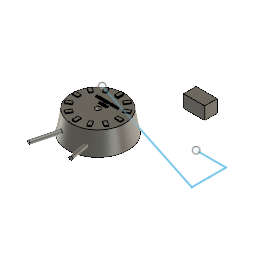
AlarmClock v1 (Autodesk Fusion 360 design; units mm, degrees)
Autodesk Fusion 360 part; units mm, degrees
(part 1 of 2)
sketch "Sketch1" plane through (0, 0, 0) normal (0, 0, 1) x (1, 0, 0)
  circle A0 centre (0, 0) radius 70.7107
  constraint coincident A0.centre origin
extrude "Extrude1" add sketch "Sketch1" along normal blind 50 draft -10 makes body 1
sketch "Sketch2" plane through (0, 0, 50) normal (0, 0, 1) x (-1, 0, 0)
  circle A0 centre (0, 0) radius 61.8943
  line L0 (3.9578, -43.206) -> (-3.9578, -43.206)
  line L1 (-3.9578, -43.206) -> (-3.9578, -56.794)
  line L2 (-3.9578, -56.794) -> (3.9578, -56.794)
  line L3 (3.9578, -56.794) -> (3.9578, -43.206)
  line L4 (3.9578, -43.206) -> (-3.9578, -56.794) construction
  line L5 (-3.9578, -43.206) -> (3.9578, -56.794) construction
  point P0 (0, -50)
  constraint horizontal L0
  constraint perpendicular L0 L1
  constraint parallel L0 L2
  constraint parallel L1 L3
  constraint coincident L4 P0
  constraint coincident L5 P0
extrude "Extrude2" add sketch "Sketch2" along normal blind 2 contours L0 L1 L2 L3 bodies 1
extrude "Extrude3" add 1 faces at (1.3193, 47.7353, 52) along direction (0, 0, 1) blind 2 separate body on bodies 1 makes body 2
pattern_circular "C-Pattern1" count 12 over 360 about axis through (0, 0, 1.75) along (0, 0, 1) of bodies 2 makes body 3 at (-24.9898, 45.9222, 52) makes body 4 at (-41.9996, 22.7251, 52) makes body 5 at (-47.7353, 1.3193, 52) makes body 6 at (-40.6804, -25.0102, 52) makes body 7 at (-25.0102, -40.6804, 52) makes body 8 at (-1.3193, -47.7353, 52) makes body 9 at (22.7251, -41.9996, 52) makes body 10 at (40.6804, -25.0102, 52) makes body 11 at (47.7353, -1.3193, 52) makes body 12 at (41.9996, 22.7251, 52) makes body 13 at (25.0102, 40.6804, 52)
sketch "Sketch3" plane through (0, 0, 50) normal (0, 0, 1) x (-1, 0, 0)
  line L0 (3.9578, -56.794) -> (-3.9578, -56.794)
  line L1 (-3.9578, -56.794) -> (-3.9578, -43.206)
  line L2 (-3.9578, -43.206) -> (3.9578, -43.206)
  line L3 (3.9578, -43.206) -> (3.9578, -56.794)
  circle A0 centre (0, 0) radius 61.8943
  circle A1 centre (0, 0) radius 6.2665
  constraint coincident A0.centre A1.centre
extrude "Extrude4" cut sketch "Sketch3" against normal blind 30 contours A1 bodies 1
sketch "Sketch4" plane through (0, 0, 50) normal (0, 0, 1) x (-1, 0, 0)
  circle A0 centre (0, 0) radius 6.2665
  line L0 (3.9578, -56.794) -> (-3.9578, -56.794)
  line L1 (-3.9578, -56.794) -> (-3.9578, -43.206)
  line L2 (-3.9578, -43.206) -> (3.9578, -43.206)
  line L3 (3.9578, -43.206) -> (3.9578, -56.794)
  circle A1 centre (0, 0) radius 61.8943
  line L4 (20, -10) -> (-20, -10)
  dimension "d12" = 5
  dimension "d13" = 5
  text T0 "NGUYEN VAN A" font "Arial" height 5 align centre spacing 1 along the path letters at x, y, angle (26.4137, -26.3233, 180) (21.3694, -26.3233, 180) (15.9362, -26.3233, 180) (10.8919, -26.3233, 180) (6.2329, -26.3233, 180) (1.574, -26.3233, 180) (-3.4703, -26.3233, 180) (-5.411, -26.3233, 180) (-10.0699, -26.3233, 180) (-14.7493, -26.3233, 180) (-19.7937, -26.3233, 180) (-21.7343, -26.3233, 180)
  text T1 "MSSV" font "Arial" height 5 align centre spacing 1 along the path L4 letters at x, y, angle (9.8977, -16.3233, 180) (4.0791, -16.3233, 180) (-0.5798, -16.3233, 180) (-5.2387, -16.3233, 180)
  constraint horizontal L4
extrude "Extrude5" add sketch "Sketch4" along normal blind 2 text T0 T1 bodies 1
sketch "Sketch5" plane through (0, 0, 50) normal (0, 0, 1) x (-1, 0, 0)
  line L0 (9.3793, -10) -> (9.3793, -15)
  line L1 (9.3793, -15) -> (8.3834, -15)
  line L2 (8.3834, -15) -> (7.1999, -11.4598)
  spline S0 degree 3 poles (7.1999, -11.4598) (7.1522, -11.3158) (7.0708, -11.0697) (6.9933, -10.8223) (6.9611, -10.7196) knots 0 0 0 0 0.045488 0.077767 0.077767 0.077767 0.077767
  spline S1 degree 3 poles (6.9611, -10.7196) (6.925, -10.832) (6.8389, -11.1) (6.7479, -11.3664) (6.6951, -11.5211) knots 0 0 0 0 0.035404 0.084451 0.084451 0.084451 0.084451
  line L3 (6.6951, -11.5211) -> (5.498, -15)
  line L4 (5.498, -15) -> (4.6078, -15)
  line L5 (4.6078, -15) -> (4.6078, -10)
  line L6 (4.6078, -10) -> (5.2456, -10)
  line L7 (5.2456, -10) -> (5.2456, -14.1849)
  line L8 (5.2456, -14.1849) -> (6.6985, -10)
  line L9 (6.6985, -10) -> (7.2954, -10)
  line L10 (7.2954, -10) -> (8.7415, -14.2565)
  line L11 (8.7415, -14.2565) -> (8.7415, -10)
  line L12 (8.7415, -10) -> (9.3793, -10)
  line L13 (-7.2067, -10) -> (-5.2694, -15)
  line L14 (-5.2694, -15) -> (-5.9857, -15)
  line L15 (-5.9857, -15) -> (-7.2851, -11.3677)
  spline S2 degree 3 poles (-7.2851, -11.3677) (-7.3345, -11.2271) (-7.4296, -10.9567) (-7.5094, -10.6814) (-7.5477, -10.5491) knots 0 0 0 0 0.04468 0.08598 0.08598 0.08598 0.08598
  spline S3 degree 3 poles (-7.5477, -10.5491) (-7.5881, -10.686) (-7.6695, -10.9616) (-7.7677, -11.2317) (-7.8172, -11.3677) knots 0 0 0 0 0.042804 0.086194 0.086194 0.086194 0.086194
  line L16 (-7.8172, -11.3677) -> (-9.1678, -15)
  line L17 (-9.1678, -15) -> (-9.8431, -15)
  line L18 (-9.8431, -15) -> (-7.8854, -10)
  line L19 (-7.8854, -10) -> (-7.2067, -10)
  line L20 (25.8817, -20) -> (25.8817, -25)
  line L21 (25.8817, -25) -> (25.2029, -25)
  line L22 (25.2029, -25) -> (22.5767, -21.0744)
  line L23 (22.5767, -21.0744) -> (22.5767, -25)
  line L24 (22.5767, -25) -> (21.9424, -25)
  line L25 (21.9424, -25) -> (21.9424, -20)
  line L26 (21.9424, -20) -> (22.6211, -20)
  line L27 (22.6211, -20) -> (25.2473, -23.9291)
  line L28 (25.2473, -23.9291) -> (25.2473, -20)
  line L29 (25.2473, -20) -> (25.8817, -20)
  line L30 (5.6804, -20) -> (5.6804, -25)
  line L31 (5.6804, -25) -> (2.0651, -25)
  line L32 (2.0651, -25) -> (2.0651, -24.41)
  line L33 (2.0651, -24.41) -> (5.0188, -24.41)
  line L34 (5.0188, -24.41) -> (5.0188, -22.8786)
  line L35 (5.0188, -22.8786) -> (2.2527, -22.8786)
  line L36 (2.2527, -22.8786) -> (2.2527, -22.292)
  line L37 (2.2527, -22.292) -> (5.0188, -22.292)
  line L38 (5.0188, -22.292) -> (5.0188, -20.59)
  line L39 (5.0188, -20.59) -> (1.9492, -20.59)
  line L40 (1.9492, -20.59) -> (1.9492, -20)
  line L41 (1.9492, -20) -> (5.6804, -20)
  line L42 (-15.2814, -20) -> (-15.2814, -25)
  line L43 (-15.2814, -25) -> (-15.9601, -25)
  line L44 (-15.9601, -25) -> (-18.5863, -21.0744)
  line L45 (-18.5863, -21.0744) -> (-18.5863, -25)
  line L46 (-18.5863, -25) -> (-19.2207, -25)
  line L47 (-19.2207, -25) -> (-19.2207, -20)
  line L48 (-19.2207, -20) -> (-18.542, -20)
  line L49 (-18.542, -20) -> (-15.9158, -23.9291)
  line L50 (-15.9158, -23.9291) -> (-15.9158, -20)
  line L51 (-15.9158, -20) -> (-15.2814, -20)
  line L52 (-21.7241, -20) -> (-23.6443, -25)
  line L53 (-23.6443, -25) -> (-24.3571, -25)
  line L54 (-24.3571, -25) -> (-26.4035, -20)
  line L55 (-26.4035, -20) -> (-25.6497, -20)
  line L56 (-25.6497, -20) -> (-25.0665, -21.5143)
  line L57 (-25.0665, -21.5143) -> (-22.9758, -21.5143)
  line L58 (-22.9758, -21.5143) -> (-22.4267, -20)
  line L59 (-22.4267, -20) -> (-21.7241, -20)
  line L60 (-7.3789, -20) -> (-5.4417, -25)
  line L61 (-5.4417, -25) -> (-6.1579, -25)
  line L62 (-6.1579, -25) -> (-7.4574, -21.3677)
  spline S4 degree 3 poles (-7.4574, -21.3677) (-7.5068, -21.2271) (-7.6019, -20.9567) (-7.6817, -20.6814) (-7.72, -20.5491) knots 0 0 0 0 0.04468 0.08598 0.08598 0.08598 0.08598
  spline S5 degree 3 poles (-7.72, -20.5491) (-7.7604, -20.686) (-7.8417, -20.9616) (-7.94, -21.2317) (-7.9894, -21.3677) knots 0 0 0 0 0.042804 0.086194 0.086194 0.086194 0.086194
  line L63 (-7.9894, -21.3677) -> (-9.34, -25)
  line L64 (-9.34, -25) -> (-10.0153, -25)
  line L65 (-10.0153, -25) -> (-8.0576, -20)
  line L66 (-8.0576, -20) -> (-7.3789, -20)
  line L67 (12.1163, -25) -> (11.4546, -25)
  line L68 (11.4546, -25) -> (11.4546, -22.1112)
  spline S6 degree 3 poles (11.4546, -22.1112) (11.4578, -21.8841) (11.4634, -21.4772) (11.5756, -21.0866) (11.6252, -20.9141) knots 0 0 0 0 0.06775 0.121395 0.121395 0.121395 0.121395
  spline S7 degree 3 poles (11.6252, -20.9141) (11.6954, -20.772) (11.8396, -20.48) (12.1047, -20.2902) (12.2408, -20.1927) knots 0 0 0 0 0.046779 0.096143 0.096143 0.096143 0.096143
  spline S8 degree 3 poles (12.2408, -20.1927) (12.4095, -20.1118) (12.7778, -19.9351) (13.1871, -19.9219) (13.4089, -19.9147) knots 0 0 0 0 0.055521 0.121246 0.121246 0.121246 0.121246
  spline S9 degree 3 poles (13.4089, -19.9147) (13.6249, -19.921) (14.0234, -19.9325) (14.3903, -20.0864) (14.5583, -20.1569) knots 0 0 0 0 0.064151 0.118358 0.118358 0.118358 0.118358
  spline S10 degree 3 poles (14.5583, -20.1569) (14.6964, -20.2462) (14.9709, -20.4236) (15.1213, -20.7136) (15.1961, -20.8578) knots 0 0 0 0 0.048411 0.096232 0.096232 0.096232 0.096232
  spline S11 degree 3 poles (15.1961, -20.8578) (15.2516, -21.0374) (15.3776, -21.445) (15.3837, -21.8722) (15.3871, -22.1112) knots 0 0 0 0 0.05613 0.12736 0.12736 0.12736 0.12736
  line L69 (15.3871, -22.1112) -> (15.3871, -25)
  line L70 (15.3871, -25) -> (14.7254, -25)
  line L71 (14.7254, -25) -> (14.7254, -22.1146)
  spline S12 degree 3 poles (14.7254, -22.1146) (14.7248, -21.9247) (14.7236, -21.5991) (14.6394, -21.2853) (14.6044, -21.1545) knots 0 0 0 0 0.056655 0.097122 0.097122 0.097122 0.097122
  spline S13 degree 3 poles (14.6044, -21.1545) (14.5565, -21.0573) (14.4601, -20.8618) (14.2792, -20.74) (14.1883, -20.6787) knots 0 0 0 0 0.0319 0.064192 0.064192 0.064192 0.064192
  spline S14 degree 3 poles (14.1883, -20.6787) (14.0806, -20.63) (13.8517, -20.5264) (13.6002, -20.5167) (13.4669, -20.5116) knots 0 0 0 0 0.035099 0.074671 0.074671 0.074671 0.074671
  spline S15 degree 3 poles (13.4669, -20.5116) (13.2507, -20.5165) (12.8685, -20.5251) (12.5604, -20.7464) (12.4267, -20.8424) knots 0 0 0 0 0.063045 0.111418 0.111418 0.111418 0.111418
  spline S16 degree 3 poles (12.4267, -20.8424) (12.337, -21.0002) (12.1147, -21.3909) (12.1157, -21.8443) (12.1163, -22.1146) knots 0 0 0 0 0.053658 0.13291 0.13291 0.13291 0.13291
  line L72 (12.1163, -22.1146) -> (12.1163, -25)
  line L73 (3.7653, -11.6064) -> (3.1412, -11.661)
  spline S17 degree 3 poles (3.1412, -11.661) (3.1236, -11.5447) (3.0906, -11.3272) (2.9844, -11.1349) (2.9349, -11.0454) knots 0 0 0 0 0.034936 0.065388 0.065388 0.065388 0.065388
  spline S18 degree 3 poles (2.9349, -11.0454) (2.8701, -10.9677) (2.7313, -10.8013) (2.5359, -10.7069) (2.4318, -10.6565) knots 0 0 0 0 0.030005 0.064234 0.064234 0.064234 0.064234
  spline S19 degree 3 poles (2.4318, -10.6565) (2.3122, -10.6133) (2.0643, -10.5236) (1.8008, -10.5135) (1.6644, -10.5082) knots 0 0 0 0 0.037908 0.078579 0.078579 0.078579 0.078579
  spline S20 degree 3 poles (1.6644, -10.5082) (1.5446, -10.5119) (1.3165, -10.5188) (1.0991, -10.5879) (0.9959, -10.6207) knots 0 0 0 0 0.035752 0.068081 0.068081 0.068081 0.068081
  spline S21 degree 3 poles (0.9959, -10.6207) (0.9073, -10.6593) (0.7411, -10.7316) (0.6207, -10.8664) (0.5645, -10.9294) knots 0 0 0 0 0.028587 0.053609 0.053609 0.053609 0.053609
  spline S22 degree 3 poles (0.5645, -10.9294) (0.5232, -10.9958) (0.4415, -11.1272) (0.4291, -11.2813) (0.4229, -11.3574) knots 0 0 0 0 0.023091 0.045667 0.045667 0.045667 0.045667
  spline S23 degree 3 poles (0.4229, -11.3574) (0.4282, -11.4329) (0.4387, -11.5816) (0.5196, -11.7068) (0.5593, -11.7684) knots 0 0 0 0 0.022304 0.043934 0.043934 0.043934 0.043934
  spline S24 degree 3 poles (0.5593, -11.7684) (0.6169, -11.8263) (0.7458, -11.9559) (0.9156, -12.0251) (1.0095, -12.0634) knots 0 0 0 0 0.024245 0.054313 0.054313 0.054313 0.054313
  spline S25 degree 3 poles (1.0095, -12.0634) (1.117, -12.0979) (1.4101, -12.1919) (1.7098, -12.2625) (1.8997, -12.3073) knots 0 0 0 0 0.033833 0.092327 0.092327 0.092327 0.092327
  spline S26 degree 3 poles (1.8997, -12.3073) (2.0971, -12.3545) (2.4273, -12.4334) (2.7394, -12.566) (2.8649, -12.6194) knots 0 0 0 0 0.060743 0.101593 0.101593 0.101593 0.101593
  spline S27 degree 3 poles (2.8649, -12.6194) (2.9749, -12.6829) (3.1835, -12.8034) (3.3296, -12.9945) (3.3987, -13.0849) knots 0 0 0 0 0.037661 0.07145 0.07145 0.07145 0.07145
  spline S28 degree 3 poles (3.3987, -13.0849) (3.4499, -13.181) (3.5537, -13.3757) (3.5674, -13.5959) (3.5744, -13.7074) knots 0 0 0 0 0.032271 0.065348 0.065348 0.065348 0.065348
  spline S29 degree 3 poles (3.5744, -13.7074) (3.565, -13.832) (3.5462, -14.0839) (3.4222, -14.3039) (3.3595, -14.4151) knots 0 0 0 0 0.037014 0.074774 0.074774 0.074774 0.074774
  spline S30 degree 3 poles (3.3595, -14.4151) (3.2774, -14.5191) (3.1075, -14.7344) (2.8599, -14.8533) (2.7319, -14.9147) knots 0 0 0 0 0.0392 0.081166 0.081166 0.081166 0.081166
  spline S31 degree 3 poles (2.7319, -14.9147) (2.588, -14.9645) (2.2909, -15.0671) (1.9766, -15.0791) (1.8145, -15.0853) knots 0 0 0 0 0.045409 0.093773 0.093773 0.093773 0.093773
  spline S32 degree 3 poles (1.8145, -15.0853) (1.6384, -15.0794) (1.3025, -15.0681) (0.985, -14.9584) (0.8339, -14.9062) knots 0 0 0 0 0.052502 0.100178 0.100178 0.100178 0.100178
  spline S33 degree 3 poles (0.8339, -14.9062) (0.7016, -14.8411) (0.4441, -14.7144) (0.2669, -14.4889) (0.1808, -14.3793) knots 0 0 0 0 0.043593 0.08488 0.08488 0.08488 0.08488
  spline S34 degree 3 poles (0.1808, -14.3793) (0.1134, -14.2584) (-0.0235, -14.013) (-0.0509, -13.7333) (-0.0648, -13.5914) knots 0 0 0 0 0.04104 0.083317 0.083317 0.083317 0.083317
  line L74 (-0.0648, -13.5914) -> (0.5696, -13.5437)
  spline S35 degree 3 poles (0.5696, -13.5437) (0.5934, -13.6891) (0.6383, -13.963) (0.8272, -14.1651) (0.9158, -14.2599) knots 0 0 0 0 0.043094 0.081155 0.081155 0.081155 0.081155
  spline S36 degree 3 poles (0.9158, -14.2599) (1.0346, -14.3303) (1.3019, -14.4886) (1.6139, -14.4973) (1.7872, -14.502) knots 0 0 0 0 0.040802 0.091768 0.091768 0.091768 0.091768
  spline S37 degree 3 poles (1.7872, -14.502) (1.9644, -14.4994) (2.275, -14.4946) (2.5458, -14.3459) (2.662, -14.2821) knots 0 0 0 0 0.052175 0.091411 0.091411 0.091411 0.091411
  spline S38 degree 3 poles (2.662, -14.2821) (2.7421, -14.207) (2.8965, -14.0621) (2.9235, -13.8526) (2.9366, -13.7517) knots 0 0 0 0 0.031819 0.061404 0.061404 0.061404 0.061404
  spline S39 degree 3 poles (2.9366, -13.7517) (2.9288, -13.6661) (2.9133, -13.4966) (2.7989, -13.3707) (2.7422, -13.3083) knots 0 0 0 0 0.025033 0.049607 0.049607 0.049607 0.049607
  spline S40 degree 3 poles (2.7422, -13.3083) (2.6289, -13.2452) (2.3176, -13.0717) (1.9674, -12.9985) (1.7445, -12.9519) knots 0 0 0 0 0.038725 0.106441 0.106441 0.106441 0.106441
  spline S41 degree 3 poles (1.7445, -12.9519) (1.5161, -12.9009) (1.1405, -12.817) (0.7793, -12.6848) (0.6378, -12.633) knots 0 0 0 0 0.070116 0.115283 0.115283 0.115283 0.115283
  spline S42 degree 3 poles (0.6378, -12.633) (0.5045, -12.5654) (0.2548, -12.4386) (0.0764, -12.2235) (-0.0068, -12.1231) knots 0 0 0 0 0.044271 0.082966 0.082966 0.082966 0.082966
  spline S43 degree 3 poles (-0.0068, -12.1231) (-0.0675, -12.015) (-0.1914, -11.7941) (-0.2069, -11.5411) (-0.2149, -11.412) knots 0 0 0 0 0.036694 0.07495 0.07495 0.07495 0.07495
  spline S44 degree 3 poles (-0.2149, -11.412) (-0.2048, -11.2801) (-0.1845, -11.0126) (-0.053, -10.7786) (0.0136, -10.66) knots 0 0 0 0 0.039172 0.079452 0.079452 0.079452 0.079452
  spline S45 degree 3 poles (0.0136, -10.66) (0.1002, -10.5479) (0.2785, -10.3169) (0.5371, -10.1809) (0.6702, -10.1108) knots 0 0 0 0 0.041948 0.086488 0.086488 0.086488 0.086488
  spline S46 degree 3 poles (0.6702, -10.1108) (0.8201, -10.0537) (1.1303, -9.9354) (1.4622, -9.9218) (1.6337, -9.9147) knots 0 0 0 0 0.047808 0.098905 0.098905 0.098905 0.098905
  spline S47 degree 3 poles (1.6337, -9.9147) (1.8436, -9.9201) (2.233, -9.9299) (2.6014, -10.0549) (2.7711, -10.1126) knots 0 0 0 0 0.062568 0.11604 0.11604 0.11604 0.11604
  spline S48 degree 3 poles (2.7711, -10.1126) (2.9152, -10.1859) (3.1996, -10.3307) (3.3946, -10.5832) (3.4908, -10.7077) knots 0 0 0 0 0.047839 0.094429 0.094429 0.094429 0.094429
  spline S49 degree 3 poles (3.4908, -10.7077) (3.5675, -10.8456) (3.7231, -11.1255) (3.7511, -11.4446) (3.7653, -11.6064) knots 0 0 0 0 0.046783 0.094914 0.094914 0.094914 0.094914
  line L75 (-0.8936, -11.6064) -> (-1.5177, -11.661)
  spline S50 degree 3 poles (-1.5177, -11.661) (-1.5353, -11.5447) (-1.5683, -11.3272) (-1.6746, -11.1349) (-1.7241, -11.0454) knots 0 0 0 0 0.034936 0.065388 0.065388 0.065388 0.065388
  spline S51 degree 3 poles (-1.7241, -11.0454) (-1.7889, -10.9677) (-1.9276, -10.8013) (-2.123, -10.7069) (-2.2271, -10.6565) knots 0 0 0 0 0.030005 0.064234 0.064234 0.064234 0.064234
  spline S52 degree 3 poles (-2.2271, -10.6565) (-2.3467, -10.6133) (-2.5946, -10.5236) (-2.8581, -10.5135) (-2.9945, -10.5082) knots 0 0 0 0 0.037908 0.078579 0.078579 0.078579 0.078579
  spline S53 degree 3 poles (-2.9945, -10.5082) (-3.1143, -10.5119) (-3.3425, -10.5188) (-3.5598, -10.5879) (-3.663, -10.6207) knots 0 0 0 0 0.035752 0.068081 0.068081 0.068081 0.068081
  spline S54 degree 3 poles (-3.663, -10.6207) (-3.7516, -10.6593) (-3.9178, -10.7316) (-4.0382, -10.8664) (-4.0945, -10.9294) knots 0 0 0 0 0.028587 0.053609 0.053609 0.053609 0.053609
  spline S55 degree 3 poles (-4.0945, -10.9294) (-4.1358, -10.9958) (-4.2174, -11.1272) (-4.2299, -11.2813) (-4.236, -11.3574) knots 0 0 0 0 0.023091 0.045667 0.045667 0.045667 0.045667
  spline S56 degree 3 poles (-4.236, -11.3574) (-4.2307, -11.4329) (-4.2202, -11.5816) (-4.1394, -11.7068) (-4.0996, -11.7684) knots 0 0 0 0 0.022304 0.043934 0.043934 0.043934 0.043934
  spline S57 degree 3 poles (-4.0996, -11.7684) (-4.0421, -11.8263) (-3.9132, -11.9559) (-3.7434, -12.0251) (-3.6494, -12.0634) knots 0 0 0 0 0.024245 0.054313 0.054313 0.054313 0.054313
  spline S58 degree 3 poles (-3.6494, -12.0634) (-3.542, -12.0979) (-3.2488, -12.1919) (-2.9491, -12.2625) (-2.7592, -12.3073) knots 0 0 0 0 0.033833 0.092327 0.092327 0.092327 0.092327
  spline S59 degree 3 poles (-2.7592, -12.3073) (-2.5618, -12.3545) (-2.2316, -12.4334) (-1.9195, -12.566) (-1.794, -12.6194) knots 0 0 0 0 0.060743 0.101593 0.101593 0.101593 0.101593
  spline S60 degree 3 poles (-1.794, -12.6194) (-1.684, -12.6829) (-1.4754, -12.8034) (-1.3293, -12.9945) (-1.2602, -13.0849) knots 0 0 0 0 0.037661 0.07145 0.07145 0.07145 0.07145
  spline S61 degree 3 poles (-1.2602, -13.0849) (-1.209, -13.181) (-1.1053, -13.3757) (-1.0915, -13.5959) (-1.0846, -13.7074) knots 0 0 0 0 0.032271 0.065348 0.065348 0.065348 0.065348
  spline S62 degree 3 poles (-1.0846, -13.7074) (-1.0939, -13.832) (-1.1127, -14.0839) (-1.2368, -14.3039) (-1.2995, -14.4151) knots 0 0 0 0 0.037014 0.074774 0.074774 0.074774 0.074774
  spline S63 degree 3 poles (-1.2995, -14.4151) (-1.3815, -14.5191) (-1.5515, -14.7344) (-1.799, -14.8533) (-1.927, -14.9147) knots 0 0 0 0 0.0392 0.081166 0.081166 0.081166 0.081166
  spline S64 degree 3 poles (-1.927, -14.9147) (-2.0709, -14.9645) (-2.3681, -15.0671) (-2.6824, -15.0791) (-2.8445, -15.0853) knots 0 0 0 0 0.045409 0.093773 0.093773 0.093773 0.093773
  spline S65 degree 3 poles (-2.8445, -15.0853) (-3.0205, -15.0794) (-3.3565, -15.0681) (-3.6739, -14.9584) (-3.825, -14.9062) knots 0 0 0 0 0.052502 0.100178 0.100178 0.100178 0.100178
  spline S66 degree 3 poles (-3.825, -14.9062) (-3.9573, -14.8411) (-4.2148, -14.7144) (-4.392, -14.4889) (-4.4782, -14.3793) knots 0 0 0 0 0.043593 0.08488 0.08488 0.08488 0.08488
  spline S67 degree 3 poles (-4.4782, -14.3793) (-4.5456, -14.2584) (-4.6824, -14.013) (-4.7098, -13.7333) (-4.7237, -13.5914) knots 0 0 0 0 0.04104 0.083317 0.083317 0.083317 0.083317
  line L76 (-4.7237, -13.5914) -> (-4.0894, -13.5437)
  spline S68 degree 3 poles (-4.0894, -13.5437) (-4.0655, -13.6891) (-4.0206, -13.963) (-3.8318, -14.1651) (-3.7432, -14.2599) knots 0 0 0 0 0.043094 0.081155 0.081155 0.081155 0.081155
  spline S69 degree 3 poles (-3.7432, -14.2599) (-3.6243, -14.3303) (-3.357, -14.4886) (-3.045, -14.4973) (-2.8718, -14.502) knots 0 0 0 0 0.040802 0.091768 0.091768 0.091768 0.091768
  spline S70 degree 3 poles (-2.8718, -14.502) (-2.6945, -14.4994) (-2.3839, -14.4946) (-2.1131, -14.3459) (-1.9969, -14.2821) knots 0 0 0 0 0.052175 0.091411 0.091411 0.091411 0.091411
  spline S71 degree 3 poles (-1.9969, -14.2821) (-1.9169, -14.207) (-1.7624, -14.0621) (-1.7354, -13.8526) (-1.7224, -13.7517) knots 0 0 0 0 0.031819 0.061404 0.061404 0.061404 0.061404
  spline S72 degree 3 poles (-1.7224, -13.7517) (-1.7302, -13.6661) (-1.7456, -13.4966) (-1.8601, -13.3707) (-1.9168, -13.3083) knots 0 0 0 0 0.025033 0.049607 0.049607 0.049607 0.049607
  spline S73 degree 3 poles (-1.9168, -13.3083) (-2.03, -13.2452) (-2.3413, -13.0717) (-2.6916, -12.9985) (-2.9144, -12.9519) knots 0 0 0 0 0.038725 0.106441 0.106441 0.106441 0.106441
  spline S74 degree 3 poles (-2.9144, -12.9519) (-3.1428, -12.9009) (-3.5184, -12.817) (-3.8796, -12.6848) (-4.0211, -12.633) knots 0 0 0 0 0.070116 0.115283 0.115283 0.115283 0.115283
  spline S75 degree 3 poles (-4.0211, -12.633) (-4.1544, -12.5654) (-4.4041, -12.4386) (-4.5825, -12.2235) (-4.6658, -12.1231) knots 0 0 0 0 0.044271 0.082966 0.082966 0.082966 0.082966
  spline S76 degree 3 poles (-4.6658, -12.1231) (-4.7264, -12.015) (-4.8504, -11.7941) (-4.8659, -11.5411) (-4.8738, -11.412) knots 0 0 0 0 0.036694 0.07495 0.07495 0.07495 0.07495
  spline S77 degree 3 poles (-4.8738, -11.412) (-4.8638, -11.2801) (-4.8434, -11.0126) (-4.7119, -10.7786) (-4.6453, -10.66) knots 0 0 0 0 0.039172 0.079452 0.079452 0.079452 0.079452
  spline S78 degree 3 poles (-4.6453, -10.66) (-4.5588, -10.5479) (-4.3804, -10.3169) (-4.1219, -10.1809) (-3.9887, -10.1108) knots 0 0 0 0 0.041948 0.086488 0.086488 0.086488 0.086488
  spline S79 degree 3 poles (-3.9887, -10.1108) (-3.8388, -10.0537) (-3.5286, -9.9354) (-3.1967, -9.9218) (-3.0252, -9.9147) knots 0 0 0 0 0.047808 0.098905 0.098905 0.098905 0.098905
  spline S80 degree 3 poles (-3.0252, -9.9147) (-2.8153, -9.9201) (-2.4259, -9.9299) (-2.0575, -10.0549) (-1.8878, -10.1126) knots 0 0 0 0 0.062568 0.11604 0.11604 0.11604 0.11604
  spline S81 degree 3 poles (-1.8878, -10.1126) (-1.7437, -10.1859) (-1.4593, -10.3307) (-1.2643, -10.5832) (-1.1681, -10.7077) knots 0 0 0 0 0.047839 0.094429 0.094429 0.094429 0.094429
  spline S82 degree 3 poles (-1.1681, -10.7077) (-1.0914, -10.8456) (-0.9358, -11.1255) (-0.9078, -11.4446) (-0.8936, -11.6064) knots 0 0 0 0 0.046783 0.094914 0.094914 0.094914 0.094914
  circle A0 centre (0, 0) radius 6.2665
  line L77 (3.9578, -56.794) -> (-3.9578, -56.794)
  line L78 (-3.9578, -56.794) -> (-3.9578, -43.206)
  line L79 (-3.9578, -43.206) -> (3.9578, -43.206)
  line L80 (3.9578, -43.206) -> (3.9578, -56.794)
  circle A1 centre (0, 0) radius 61.8943
  line L81 (1.042, -20) -> (1.042, -25)
  line L82 (1.042, -25) -> (0.3632, -25)
  line L83 (0.3632, -25) -> (-2.263, -21.0744)
  line L84 (-2.263, -21.0744) -> (-2.263, -25)
  line L85 (-2.263, -25) -> (-2.8973, -25)
  line L86 (-2.8973, -25) -> (-2.8973, -20)
  line L87 (-2.8973, -20) -> (-2.2186, -20)
  line L88 (-2.2186, -20) -> (0.4076, -23.9291)
  line L89 (0.4076, -23.9291) -> (0.4076, -20)
  line L90 (0.4076, -20) -> (1.042, -20)
  line L91 (18.4908, -21.9611) -> (18.4908, -22.5477)
  line L92 (18.4908, -22.5477) -> (16.3728, -22.5512)
  line L93 (16.3728, -22.5512) -> (16.3728, -20.6958)
  spline S83 degree 3 poles (16.3728, -20.6958) (16.5339, -20.5753) (16.8467, -20.3412) (17.2051, -20.1861) (17.3789, -20.1108) knots 0 0 0 0 0.060121 0.116737 0.116737 0.116737 0.116737
  spline S84 degree 3 poles (17.3789, -20.1108) (17.5525, -20.0536) (17.8983, -19.9397) (18.2619, -19.923) (18.443, -19.9147) knots 0 0 0 0 0.054544 0.108655 0.108655 0.108655 0.108655
  spline S85 degree 3 poles (18.443, -19.9147) (18.6808, -19.9267) (19.1465, -19.9502) (19.573, -20.1382) (19.7817, -20.2302) knots 0 0 0 0 0.070743 0.13857 0.13857 0.13857 0.13857
  spline S86 degree 3 poles (19.7817, -20.2302) (19.9699, -20.3468) (20.345, -20.5791) (20.5757, -20.9552) (20.6907, -21.1426) knots 0 0 0 0 0.065413 0.130387 0.130387 0.130387 0.130387
  spline S87 degree 3 poles (20.6907, -21.1426) (20.7802, -21.3502) (20.9637, -21.7758) (20.9861, -22.2389) (20.9976, -22.4761) knots 0 0 0 0 0.067246 0.137838 0.137838 0.137838 0.137838
  spline S88 degree 3 poles (20.9976, -22.4761) (20.9854, -22.7143) (20.9612, -23.186) (20.7814, -23.6225) (20.6924, -23.8387) knots 0 0 0 0 0.070969 0.140541 0.140541 0.140541 0.140541
  spline S89 degree 3 poles (20.6924, -23.8387) (20.5815, -24.0349) (20.3644, -24.4192) (19.995, -24.6603) (19.8141, -24.7783) knots 0 0 0 0 0.066513 0.130304 0.130304 0.130304 0.130304
  spline S90 degree 3 poles (19.8141, -24.7783) (19.6117, -24.8678) (19.1915, -25.0535) (18.7322, -25.0744) (18.4942, -25.0853) knots 0 0 0 0 0.065806 0.136568 0.136568 0.136568 0.136568
  spline S91 degree 3 poles (18.4942, -25.0853) (18.3206, -25.079) (17.9852, -25.067) (17.6671, -24.9608) (17.5136, -24.9096) knots 0 0 0 0 0.051815 0.100075 0.100075 0.100075 0.100075
  spline S92 degree 3 poles (17.5136, -24.9096) (17.3774, -24.8477) (17.1162, -24.7291) (16.9202, -24.5202) (16.8264, -24.4202) knots 0 0 0 0 0.044386 0.085101 0.085101 0.085101 0.085101
  spline S93 degree 3 poles (16.8264, -24.4202) (16.7471, -24.3026) (16.5772, -24.0504) (16.4928, -23.7578) (16.4478, -23.6016) knots 0 0 0 0 0.042276 0.09068 0.09068 0.09068 0.09068
  line L94 (16.4478, -23.6016) -> (17.0447, -23.4379)
  spline S94 degree 3 poles (17.0447, -23.4379) (17.0814, -23.5542) (17.1484, -23.7667) (17.2695, -23.9536) (17.3244, -24.0382) knots 0 0 0 0 0.036366 0.06649 0.06649 0.06649 0.06649
  spline S95 degree 3 poles (17.3244, -24.0382) (17.3885, -24.1084) (17.5241, -24.2566) (17.706, -24.3425) (17.8018, -24.3878) knots 0 0 0 0 0.028251 0.059684 0.059684 0.059684 0.059684
  spline S96 degree 3 poles (17.8018, -24.3878) (17.9099, -24.4261) (18.1328, -24.505) (18.3691, -24.5143) (18.4908, -24.5191) knots 0 0 0 0 0.034191 0.070493 0.070493 0.070493 0.070493
  spline S97 degree 3 poles (18.4908, -24.5191) (18.6331, -24.5149) (18.9015, -24.5069) (19.1558, -24.4212) (19.2752, -24.381) knots 0 0 0 0 0.042433 0.080041 0.080041 0.080041 0.080041
  spline S98 degree 3 poles (19.2752, -24.381) (19.3786, -24.3331) (19.5766, -24.2412) (19.7338, -24.09) (19.809, -24.0177) knots 0 0 0 0 0.033893 0.064964 0.064964 0.064964 0.064964
  spline S99 degree 3 poles (19.809, -24.0177) (19.8727, -23.9413) (19.9989, -23.7898) (20.0829, -23.6115) (20.1245, -23.5232) knots 0 0 0 0 0.029716 0.058873 0.058873 0.058873 0.058873
  spline S100 degree 3 poles (20.1245, -23.5232) (20.1802, -23.3636) (20.2939, -23.0378) (20.3082, -22.6929) (20.3155, -22.5171) knots 0 0 0 0 0.050423 0.102909 0.102909 0.102909 0.102909
  spline S101 degree 3 poles (20.3155, -22.5171) (20.309, -22.3097) (20.2969, -21.9229) (20.1523, -21.5646) (20.0853, -21.3984) knots 0 0 0 0 0.061661 0.11501 0.11501 0.11501 0.11501
  spline S102 degree 3 poles (20.0853, -21.3984) (20.0004, -21.2582) (19.8319, -20.9802) (19.5533, -20.8129) (19.4151, -20.7299) knots 0 0 0 0 0.048346 0.095938 0.095938 0.095938 0.095938
  spline S103 degree 3 poles (19.4151, -20.7299) (19.266, -20.6662) (18.9673, -20.5387) (18.643, -20.5206) (18.4806, -20.5116) knots 0 0 0 0 0.048225 0.096624 0.096624 0.096624 0.096624
  spline S104 degree 3 poles (18.4806, -20.5116) (18.3377, -20.5187) (18.05, -20.5329) (17.7783, -20.6288) (17.6415, -20.677) knots 0 0 0 0 0.042663 0.08592 0.08592 0.08592 0.08592
  spline S105 degree 3 poles (17.6415, -20.677) (17.5185, -20.7287) (17.2973, -20.8217) (17.1058, -20.966) (17.0208, -21.03) knots 0 0 0 0 0.039837 0.071651 0.071651 0.071651 0.071651
  line L95 (17.0208, -21.03) -> (17.0208, -21.9611)
  line L96 (17.0208, -21.9611) -> (18.4908, -21.9611)
  line L97 (8.9444, -20) -> (8.9444, -22.118)
  line L98 (8.9444, -22.118) -> (10.8714, -25)
  line L99 (10.8714, -25) -> (10.0665, -25)
  line L100 (10.0665, -25) -> (9.0808, -23.4925)
  spline S106 degree 3 poles (9.0808, -23.4925) (8.9918, -23.3522) (8.8156, -23.0744) (8.6531, -22.7883) (8.5726, -22.6467) knots 0 0 0 0 0.049828 0.098689 0.098689 0.098689 0.098689
  spline S107 degree 3 poles (8.5726, -22.6467) (8.4906, -22.7862) (8.3151, -23.0846) (8.127, -23.3753) (8.0269, -23.53) knots 0 0 0 0 0.048563 0.103842 0.103842 0.103842 0.103842
  line L101 (8.0269, -23.53) -> (7.0583, -25)
  line L102 (7.0583, -25) -> (6.2875, -25)
  line L103 (6.2875, -25) -> (8.2827, -22.118)
  line L104 (8.2827, -22.118) -> (8.2827, -20)
  line L105 (8.2827, -20) -> (8.9444, -20)
  line L106 (-10.0597, -20) -> (-11.9799, -25)
  line L107 (-11.9799, -25) -> (-12.6927, -25)
  line L108 (-12.6927, -25) -> (-14.7391, -20)
  line L109 (-14.7391, -20) -> (-13.9853, -20)
  line L110 (-13.9853, -20) -> (-13.4021, -21.5143)
  line L111 (-13.4021, -21.5143) -> (-11.3114, -21.5143)
  line L112 (-11.3114, -21.5143) -> (-10.7623, -20)
  line L113 (-10.7623, -20) -> (-10.0597, -20)
  circle A2 centre (-130, -50) radius 4.8024
extrude "Extrude6" add sketch "Sketch5" along normal blind 60 separate body contours A2 makes body 14
move_body "Move2" bodies 14 to x (-0.336824, 0.059391, 0.939693) y (-0.881204, 0.331707, -0.336824) z (-0.331707, -0.941511, -0.059391) at (79.2792, -38.2395, -81.1706)
sketch "Sketch6" plane through (0, 0, 0) normal (0, 1, 0) x (1, 0, 0)
sketch "Sketch7" plane through (0, 0, 50) normal (0, 0, 1) x (-1, 0, 0)
  line L0 (9.3793, -10) -> (9.3793, -15)
  line L1 (9.3793, -15) -> (8.3834, -15)
  line L2 (8.3834, -15) -> (7.1999, -11.4598)
  spline S0 degree 3 poles (7.1999, -11.4598) (7.1522, -11.3158) (7.0708, -11.0697) (6.9933, -10.8223) (6.9611, -10.7196) knots 0 0 0 0 0.045488 0.077767 0.077767 0.077767 0.077767
  spline S1 degree 3 poles (6.9611, -10.7196) (6.925, -10.832) (6.8389, -11.1) (6.7479, -11.3664) (6.6951, -11.5211) knots 0 0 0 0 0.035404 0.084451 0.084451 0.084451 0.084451
  line L3 (6.6951, -11.5211) -> (5.498, -15)
  line L4 (5.498, -15) -> (4.6078, -15)
  line L5 (4.6078, -15) -> (4.6078, -10)
  line L6 (4.6078, -10) -> (5.2456, -10)
  line L7 (5.2456, -10) -> (5.2456, -14.1849)
  line L8 (5.2456, -14.1849) -> (6.6985, -10)
  line L9 (6.6985, -10) -> (7.2954, -10)
  line L10 (7.2954, -10) -> (8.7415, -14.2565)
  line L11 (8.7415, -14.2565) -> (8.7415, -10)
  line L12 (8.7415, -10) -> (9.3793, -10)
  line L13 (-7.2067, -10) -> (-5.2694, -15)
  line L14 (-5.2694, -15) -> (-5.9857, -15)
  line L15 (-5.9857, -15) -> (-7.2851, -11.3677)
  spline S2 degree 3 poles (-7.2851, -11.3677) (-7.3345, -11.2271) (-7.4296, -10.9567) (-7.5094, -10.6814) (-7.5477, -10.5491) knots 0 0 0 0 0.04468 0.08598 0.08598 0.08598 0.08598
  spline S3 degree 3 poles (-7.5477, -10.5491) (-7.5881, -10.686) (-7.6695, -10.9616) (-7.7677, -11.2317) (-7.8172, -11.3677) knots 0 0 0 0 0.042804 0.086194 0.086194 0.086194 0.086194
  line L16 (-7.8172, -11.3677) -> (-9.1678, -15)
  line L17 (-9.1678, -15) -> (-9.8431, -15)
  line L18 (-9.8431, -15) -> (-7.8854, -10)
  line L19 (-7.8854, -10) -> (-7.2067, -10)
  line L20 (25.8817, -20) -> (25.8817, -25)
  line L21 (25.8817, -25) -> (25.2029, -25)
  line L22 (25.2029, -25) -> (22.5767, -21.0744)
  line L23 (22.5767, -21.0744) -> (22.5767, -25)
  line L24 (22.5767, -25) -> (21.9424, -25)
  line L25 (21.9424, -25) -> (21.9424, -20)
  line L26 (21.9424, -20) -> (22.6211, -20)
  line L27 (22.6211, -20) -> (25.2473, -23.9291)
  line L28 (25.2473, -23.9291) -> (25.2473, -20)
  line L29 (25.2473, -20) -> (25.8817, -20)
  line L30 (5.6804, -20) -> (5.6804, -25)
  line L31 (5.6804, -25) -> (2.0651, -25)
  line L32 (2.0651, -25) -> (2.0651, -24.41)
  line L33 (2.0651, -24.41) -> (5.0188, -24.41)
  line L34 (5.0188, -24.41) -> (5.0188, -22.8786)
  line L35 (5.0188, -22.8786) -> (2.2527, -22.8786)
  line L36 (2.2527, -22.8786) -> (2.2527, -22.292)
  line L37 (2.2527, -22.292) -> (5.0188, -22.292)
  line L38 (5.0188, -22.292) -> (5.0188, -20.59)
  line L39 (5.0188, -20.59) -> (1.9492, -20.59)
  line L40 (1.9492, -20.59) -> (1.9492, -20)
  line L41 (1.9492, -20) -> (5.6804, -20)
  line L42 (-15.2814, -20) -> (-15.2814, -25)
  line L43 (-15.2814, -25) -> (-15.9601, -25)
  line L44 (-15.9601, -25) -> (-18.5863, -21.0744)
  line L45 (-18.5863, -21.0744) -> (-18.5863, -25)
  line L46 (-18.5863, -25) -> (-19.2207, -25)
  line L47 (-19.2207, -25) -> (-19.2207, -20)
  line L48 (-19.2207, -20) -> (-18.542, -20)
  line L49 (-18.542, -20) -> (-15.9158, -23.9291)
  line L50 (-15.9158, -23.9291) -> (-15.9158, -20)
  line L51 (-15.9158, -20) -> (-15.2814, -20)
  line L52 (-21.7241, -20) -> (-23.6443, -25)
  line L53 (-23.6443, -25) -> (-24.3571, -25)
  line L54 (-24.3571, -25) -> (-26.4035, -20)
  line L55 (-26.4035, -20) -> (-25.6497, -20)
  line L56 (-25.6497, -20) -> (-25.0665, -21.5143)
  line L57 (-25.0665, -21.5143) -> (-22.9758, -21.5143)
  line L58 (-22.9758, -21.5143) -> (-22.4267, -20)
  line L59 (-22.4267, -20) -> (-21.7241, -20)
  line L60 (-7.3789, -20) -> (-5.4417, -25)
  line L61 (-5.4417, -25) -> (-6.1579, -25)
  line L62 (-6.1579, -25) -> (-7.4574, -21.3677)
  spline S4 degree 3 poles (-7.4574, -21.3677) (-7.5068, -21.2271) (-7.6019, -20.9567) (-7.6817, -20.6814) (-7.72, -20.5491) knots 0 0 0 0 0.04468 0.08598 0.08598 0.08598 0.08598
  spline S5 degree 3 poles (-7.72, -20.5491) (-7.7604, -20.686) (-7.8417, -20.9616) (-7.94, -21.2317) (-7.9894, -21.3677) knots 0 0 0 0 0.042804 0.086194 0.086194 0.086194 0.086194
  line L63 (-7.9894, -21.3677) -> (-9.34, -25)
  line L64 (-9.34, -25) -> (-10.0153, -25)
  line L65 (-10.0153, -25) -> (-8.0576, -20)
  line L66 (-8.0576, -20) -> (-7.3789, -20)
  line L67 (12.1163, -25) -> (11.4546, -25)
  line L68 (11.4546, -25) -> (11.4546, -22.1112)
  spline S6 degree 3 poles (11.4546, -22.1112) (11.4578, -21.8841) (11.4634, -21.4772) (11.5756, -21.0866) (11.6252, -20.9141) knots 0 0 0 0 0.06775 0.121395 0.121395 0.121395 0.121395
  spline S7 degree 3 poles (11.6252, -20.9141) (11.6954, -20.772) (11.8396, -20.48) (12.1047, -20.2902) (12.2408, -20.1927) knots 0 0 0 0 0.046779 0.096143 0.096143 0.096143 0.096143
  spline S8 degree 3 poles (12.2408, -20.1927) (12.4095, -20.1118) (12.7778, -19.9351) (13.1871, -19.9219) (13.4089, -19.9147) knots 0 0 0 0 0.055521 0.121246 0.121246 0.121246 0.121246
  spline S9 degree 3 poles (13.4089, -19.9147) (13.6249, -19.921) (14.0234, -19.9325) (14.3903, -20.0864) (14.5583, -20.1569) knots 0 0 0 0 0.064151 0.118358 0.118358 0.118358 0.118358
  spline S10 degree 3 poles (14.5583, -20.1569) (14.6964, -20.2462) (14.9709, -20.4236) (15.1213, -20.7136) (15.1961, -20.8578) knots 0 0 0 0 0.048411 0.096232 0.096232 0.096232 0.096232
  spline S11 degree 3 poles (15.1961, -20.8578) (15.2516, -21.0374) (15.3776, -21.445) (15.3837, -21.8722) (15.3871, -22.1112) knots 0 0 0 0 0.05613 0.12736 0.12736 0.12736 0.12736
  line L69 (15.3871, -22.1112) -> (15.3871, -25)
  line L70 (15.3871, -25) -> (14.7254, -25)
  line L71 (14.7254, -25) -> (14.7254, -22.1146)
  spline S12 degree 3 poles (14.7254, -22.1146) (14.7248, -21.9247) (14.7236, -21.5991) (14.6394, -21.2853) (14.6044, -21.1545) knots 0 0 0 0 0.056655 0.097122 0.097122 0.097122 0.097122
  spline S13 degree 3 poles (14.6044, -21.1545) (14.5565, -21.0573) (14.4601, -20.8618) (14.2792, -20.74) (14.1883, -20.6787) knots 0 0 0 0 0.0319 0.064192 0.064192 0.064192 0.064192
  spline S14 degree 3 poles (14.1883, -20.6787) (14.0806, -20.63) (13.8517, -20.5264) (13.6002, -20.5167) (13.4669, -20.5116) knots 0 0 0 0 0.035099 0.074671 0.074671 0.074671 0.074671
  spline S15 degree 3 poles (13.4669, -20.5116) (13.2507, -20.5165) (12.8685, -20.5251) (12.5604, -20.7464) (12.4267, -20.8424) knots 0 0 0 0 0.063045 0.111418 0.111418 0.111418 0.111418
  spline S16 degree 3 poles (12.4267, -20.8424) (12.337, -21.0002) (12.1147, -21.3909) (12.1157, -21.8443) (12.1163, -22.1146) knots 0 0 0 0 0.053658 0.13291 0.13291 0.13291 0.13291
  line L72 (12.1163, -22.1146) -> (12.1163, -25)
  line L73 (3.7653, -11.6064) -> (3.1412, -11.661)
  spline S17 degree 3 poles (3.1412, -11.661) (3.1236, -11.5447) (3.0906, -11.3272) (2.9844, -11.1349) (2.9349, -11.0454) knots 0 0 0 0 0.034936 0.065388 0.065388 0.065388 0.065388
  spline S18 degree 3 poles (2.9349, -11.0454) (2.8701, -10.9677) (2.7313, -10.8013) (2.5359, -10.7069) (2.4318, -10.6565) knots 0 0 0 0 0.030005 0.064234 0.064234 0.064234 0.064234
  spline S19 degree 3 poles (2.4318, -10.6565) (2.3122, -10.6133) (2.0643, -10.5236) (1.8008, -10.5135) (1.6644, -10.5082) knots 0 0 0 0 0.037908 0.078579 0.078579 0.078579 0.078579
  spline S20 degree 3 poles (1.6644, -10.5082) (1.5446, -10.5119) (1.3165, -10.5188) (1.0991, -10.5879) (0.9959, -10.6207) knots 0 0 0 0 0.035752 0.068081 0.068081 0.068081 0.068081
  spline S21 degree 3 poles (0.9959, -10.6207) (0.9073, -10.6593) (0.7411, -10.7316) (0.6207, -10.8664) (0.5645, -10.9294) knots 0 0 0 0 0.028587 0.053609 0.053609 0.053609 0.053609
  spline S22 degree 3 poles (0.5645, -10.9294) (0.5232, -10.9958) (0.4415, -11.1272) (0.4291, -11.2813) (0.4229, -11.3574) knots 0 0 0 0 0.023091 0.045667 0.045667 0.045667 0.045667
  spline S23 degree 3 poles (0.4229, -11.3574) (0.4282, -11.4329) (0.4387, -11.5816) (0.5196, -11.7068) (0.5593, -11.7684) knots 0 0 0 0 0.022304 0.043934 0.043934 0.043934 0.043934
  spline S24 degree 3 poles (0.5593, -11.7684) (0.6169, -11.8263) (0.7458, -11.9559) (0.9156, -12.0251) (1.0095, -12.0634) knots 0 0 0 0 0.024245 0.054313 0.054313 0.054313 0.054313
  spline S25 degree 3 poles (1.0095, -12.0634) (1.117, -12.0979) (1.4101, -12.1919) (1.7098, -12.2625) (1.8997, -12.3073) knots 0 0 0 0 0.033833 0.092327 0.092327 0.092327 0.092327
  spline S26 degree 3 poles (1.8997, -12.3073) (2.0971, -12.3545) (2.4273, -12.4334) (2.7394, -12.566) (2.8649, -12.6194) knots 0 0 0 0 0.060743 0.101593 0.101593 0.101593 0.101593
  spline S27 degree 3 poles (2.8649, -12.6194) (2.9749, -12.6829) (3.1835, -12.8034) (3.3296, -12.9945) (3.3987, -13.0849) knots 0 0 0 0 0.037661 0.07145 0.07145 0.07145 0.07145
  spline S28 degree 3 poles (3.3987, -13.0849) (3.4499, -13.181) (3.5537, -13.3757) (3.5674, -13.5959) (3.5744, -13.7074) knots 0 0 0 0 0.032271 0.065348 0.065348 0.065348 0.065348
  spline S29 degree 3 poles (3.5744, -13.7074) (3.565, -13.832) (3.5462, -14.0839) (3.4222, -14.3039) (3.3595, -14.4151) knots 0 0 0 0 0.037014 0.074774 0.074774 0.074774 0.074774
  spline S30 degree 3 poles (3.3595, -14.4151) (3.2774, -14.5191) (3.1075, -14.7344) (2.8599, -14.8533) (2.7319, -14.9147) knots 0 0 0 0 0.0392 0.081166 0.081166 0.081166 0.081166
  spline S31 degree 3 poles (2.7319, -14.9147) (2.588, -14.9645) (2.2909, -15.0671) (1.9766, -15.0791) (1.8145, -15.0853) knots 0 0 0 0 0.045409 0.093773 0.093773 0.093773 0.093773
  spline S32 degree 3 poles (1.8145, -15.0853) (1.6384, -15.0794) (1.3025, -15.0681) (0.985, -14.9584) (0.8339, -14.9062) knots 0 0 0 0 0.052502 0.100178 0.100178 0.100178 0.100178
  spline S33 degree 3 poles (0.8339, -14.9062) (0.7016, -14.8411) (0.4441, -14.7144) (0.2669, -14.4889) (0.1808, -14.3793) knots 0 0 0 0 0.043593 0.08488 0.08488 0.08488 0.08488
  spline S34 degree 3 poles (0.1808, -14.3793) (0.1134, -14.2584) (-0.0235, -14.013) (-0.0509, -13.7333) (-0.0648, -13.5914) knots 0 0 0 0 0.04104 0.083317 0.083317 0.083317 0.083317
  line L74 (-0.0648, -13.5914) -> (0.5696, -13.5437)
  spline S35 degree 3 poles (0.5696, -13.5437) (0.5934, -13.6891) (0.6383, -13.963) (0.8272, -14.1651) (0.9158, -14.2599) knots 0 0 0 0 0.043094 0.081155 0.081155 0.081155 0.081155
  spline S36 degree 3 poles (0.9158, -14.2599) (1.0346, -14.3303) (1.3019, -14.4886) (1.6139, -14.4973) (1.7872, -14.502) knots 0 0 0 0 0.040802 0.091768 0.091768 0.091768 0.091768
  spline S37 degree 3 poles (1.7872, -14.502) (1.9644, -14.4994) (2.275, -14.4946) (2.5458, -14.3459) (2.662, -14.2821) knots 0 0 0 0 0.052175 0.091411 0.091411 0.091411 0.091411
  spline S38 degree 3 poles (2.662, -14.2821) (2.7421, -14.207) (2.8965, -14.0621) (2.9235, -13.8526) (2.9366, -13.7517) knots 0 0 0 0 0.031819 0.061404 0.061404 0.061404 0.061404
  spline S39 degree 3 poles (2.9366, -13.7517) (2.9288, -13.6661) (2.9133, -13.4966) (2.7989, -13.3707) (2.7422, -13.3083) knots 0 0 0 0 0.025033 0.049607 0.049607 0.049607 0.049607
  spline S40 degree 3 poles (2.7422, -13.3083) (2.6289, -13.2452) (2.3176, -13.0717) (1.9674, -12.9985) (1.7445, -12.9519) knots 0 0 0 0 0.038725 0.106441 0.106441 0.106441 0.106441
  spline S41 degree 3 poles (1.7445, -12.9519) (1.5161, -12.9009) (1.1405, -12.817) (0.7793, -12.6848) (0.6378, -12.633) knots 0 0 0 0 0.070116 0.115283 0.115283 0.115283 0.115283
  spline S42 degree 3 poles (0.6378, -12.633) (0.5045, -12.5654) (0.2548, -12.4386) (0.0764, -12.2235) (-0.0068, -12.1231) knots 0 0 0 0 0.044271 0.082966 0.082966 0.082966 0.082966
  spline S43 degree 3 poles (-0.0068, -12.1231) (-0.0675, -12.015) (-0.1914, -11.7941) (-0.2069, -11.5411) (-0.2149, -11.412) knots 0 0 0 0 0.036694 0.07495 0.07495 0.07495 0.07495
  spline S44 degree 3 poles (-0.2149, -11.412) (-0.2048, -11.2801) (-0.1845, -11.0126) (-0.053, -10.7786) (0.0136, -10.66) knots 0 0 0 0 0.039172 0.079452 0.079452 0.079452 0.079452
  spline S45 degree 3 poles (0.0136, -10.66) (0.1002, -10.5479) (0.2785, -10.3169) (0.5371, -10.1809) (0.6702, -10.1108) knots 0 0 0 0 0.041948 0.086488 0.086488 0.086488 0.086488
  spline S46 degree 3 poles (0.6702, -10.1108) (0.8201, -10.0537) (1.1303, -9.9354) (1.4622, -9.9218) (1.6337, -9.9147) knots 0 0 0 0 0.047808 0.098905 0.098905 0.098905 0.098905
  spline S47 degree 3 poles (1.6337, -9.9147) (1.8436, -9.9201) (2.233, -9.9299) (2.6014, -10.0549) (2.7711, -10.1126) knots 0 0 0 0 0.062568 0.11604 0.11604 0.11604 0.11604
  spline S48 degree 3 poles (2.7711, -10.1126) (2.9152, -10.1859) (3.1996, -10.3307) (3.3946, -10.5832) (3.4908, -10.7077) knots 0 0 0 0 0.047839 0.094429 0.094429 0.094429 0.094429
  spline S49 degree 3 poles (3.4908, -10.7077) (3.5675, -10.8456) (3.7231, -11.1255) (3.7511, -11.4446) (3.7653, -11.6064) knots 0 0 0 0 0.046783 0.094914 0.094914 0.094914 0.094914
  line L75 (-0.8936, -11.6064) -> (-1.5177, -11.661)
  spline S50 degree 3 poles (-1.5177, -11.661) (-1.5353, -11.5447) (-1.5683, -11.3272) (-1.6746, -11.1349) (-1.7241, -11.0454) knots 0 0 0 0 0.034936 0.065388 0.065388 0.065388 0.065388
  spline S51 degree 3 poles (-1.7241, -11.0454) (-1.7889, -10.9677) (-1.9276, -10.8013) (-2.123, -10.7069) (-2.2271, -10.6565) knots 0 0 0 0 0.030005 0.064234 0.064234 0.064234 0.064234
  spline S52 degree 3 poles (-2.2271, -10.6565) (-2.3467, -10.6133) (-2.5946, -10.5236) (-2.8581, -10.5135) (-2.9945, -10.5082) knots 0 0 0 0 0.037908 0.078579 0.078579 0.078579 0.078579
  spline S53 degree 3 poles (-2.9945, -10.5082) (-3.1143, -10.5119) (-3.3425, -10.5188) (-3.5598, -10.5879) (-3.663, -10.6207) knots 0 0 0 0 0.035752 0.068081 0.068081 0.068081 0.068081
  spline S54 degree 3 poles (-3.663, -10.6207) (-3.7516, -10.6593) (-3.9178, -10.7316) (-4.0382, -10.8664) (-4.0945, -10.9294) knots 0 0 0 0 0.028587 0.053609 0.053609 0.053609 0.053609
  spline S55 degree 3 poles (-4.0945, -10.9294) (-4.1358, -10.9958) (-4.2174, -11.1272) (-4.2299, -11.2813) (-4.236, -11.3574) knots 0 0 0 0 0.023091 0.045667 0.045667 0.045667 0.045667
  spline S56 degree 3 poles (-4.236, -11.3574) (-4.2307, -11.4329) (-4.2202, -11.5816) (-4.1394, -11.7068) (-4.0996, -11.7684) knots 0 0 0 0 0.022304 0.043934 0.043934 0.043934 0.043934
  spline S57 degree 3 poles (-4.0996, -11.7684) (-4.0421, -11.8263) (-3.9132, -11.9559) (-3.7434, -12.0251) (-3.6494, -12.0634) knots 0 0 0 0 0.024245 0.054313 0.054313 0.054313 0.054313
  spline S58 degree 3 poles (-3.6494, -12.0634) (-3.542, -12.0979) (-3.2488, -12.1919) (-2.9491, -12.2625) (-2.7592, -12.3073) knots 0 0 0 0 0.033833 0.092327 0.092327 0.092327 0.092327
  spline S59 degree 3 poles (-2.7592, -12.3073) (-2.5618, -12.3545) (-2.2316, -12.4334) (-1.9195, -12.566) (-1.794, -12.6194) knots 0 0 0 0 0.060743 0.101593 0.101593 0.101593 0.101593
  spline S60 degree 3 poles (-1.794, -12.6194) (-1.684, -12.6829) (-1.4754, -12.8034) (-1.3293, -12.9945) (-1.2602, -13.0849) knots 0 0 0 0 0.037661 0.07145 0.07145 0.07145 0.07145
  spline S61 degree 3 poles (-1.2602, -13.0849) (-1.209, -13.181) (-1.1053, -13.3757) (-1.0915, -13.5959) (-1.0846, -13.7074) knots 0 0 0 0 0.032271 0.065348 0.065348 0.065348 0.065348
  spline S62 degree 3 poles (-1.0846, -13.7074) (-1.0939, -13.832) (-1.1127, -14.0839) (-1.2368, -14.3039) (-1.2995, -14.4151) knots 0 0 0 0 0.037014 0.074774 0.074774 0.074774 0.074774
  spline S63 degree 3 poles (-1.2995, -14.4151) (-1.3815, -14.5191) (-1.5515, -14.7344) (-1.799, -14.8533) (-1.927, -14.9147) knots 0 0 0 0 0.0392 0.081166 0.081166 0.081166 0.081166
  spline S64 degree 3 poles (-1.927, -14.9147) (-2.0709, -14.9645) (-2.3681, -15.0671) (-2.6824, -15.0791) (-2.8445, -15.0853) knots 0 0 0 0 0.045409 0.093773 0.093773 0.093773 0.093773
  spline S65 degree 3 poles (-2.8445, -15.0853) (-3.0205, -15.0794) (-3.3565, -15.0681) (-3.6739, -14.9584) (-3.825, -14.9062) knots 0 0 0 0 0.052502 0.100178 0.100178 0.100178 0.100178
  spline S66 degree 3 poles (-3.825, -14.9062) (-3.9573, -14.8411) (-4.2148, -14.7144) (-4.392, -14.4889) (-4.4782, -14.3793) knots 0 0 0 0 0.043593 0.08488 0.08488 0.08488 0.08488
  spline S67 degree 3 poles (-4.4782, -14.3793) (-4.5456, -14.2584) (-4.6824, -14.013) (-4.7098, -13.7333) (-4.7237, -13.5914) knots 0 0 0 0 0.04104 0.083317 0.083317 0.083317 0.083317
  line L76 (-4.7237, -13.5914) -> (-4.0894, -13.5437)
  spline S68 degree 3 poles (-4.0894, -13.5437) (-4.0655, -13.6891) (-4.0206, -13.963) (-3.8318, -14.1651) (-3.7432, -14.2599) knots 0 0 0 0 0.043094 0.081155 0.081155 0.081155 0.081155
  spline S69 degree 3 poles (-3.7432, -14.2599) (-3.6243, -14.3303) (-3.357, -14.4886) (-3.045, -14.4973) (-2.8718, -14.502) knots 0 0 0 0 0.040802 0.091768 0.091768 0.091768 0.091768
  spline S70 degree 3 poles (-2.8718, -14.502) (-2.6945, -14.4994) (-2.3839, -14.4946) (-2.1131, -14.3459) (-1.9969, -14.2821) knots 0 0 0 0 0.052175 0.091411 0.091411 0.091411 0.091411
  spline S71 degree 3 poles (-1.9969, -14.2821) (-1.9169, -14.207) (-1.7624, -14.0621) (-1.7354, -13.8526) (-1.7224, -13.7517) knots 0 0 0 0 0.031819 0.061404 0.061404 0.061404 0.061404
  spline S72 degree 3 poles (-1.7224, -13.7517) (-1.7302, -13.6661) (-1.7456, -13.4966) (-1.8601, -13.3707) (-1.9168, -13.3083) knots 0 0 0 0 0.025033 0.049607 0.049607 0.049607 0.049607
  spline S73 degree 3 poles (-1.9168, -13.3083) (-2.03, -13.2452) (-2.3413, -13.0717) (-2.6916, -12.9985) (-2.9144, -12.9519) knots 0 0 0 0 0.038725 0.106441 0.106441 0.106441 0.106441
  spline S74 degree 3 poles (-2.9144, -12.9519) (-3.1428, -12.9009) (-3.5184, -12.817) (-3.8796, -12.6848) (-4.0211, -12.633) knots 0 0 0 0 0.070116 0.115283 0.115283 0.115283 0.115283
  spline S75 degree 3 poles (-4.0211, -12.633) (-4.1544, -12.5654) (-4.4041, -12.4386) (-4.5825, -12.2235) (-4.6658, -12.1231) knots 0 0 0 0 0.044271 0.082966 0.082966 0.082966 0.082966
  spline S76 degree 3 poles (-4.6658, -12.1231) (-4.7264, -12.015) (-4.8504, -11.7941) (-4.8659, -11.5411) (-4.8738, -11.412) knots 0 0 0 0 0.036694 0.07495 0.07495 0.07495 0.07495
  spline S77 degree 3 poles (-4.8738, -11.412) (-4.8638, -11.2801) (-4.8434, -11.0126) (-4.7119, -10.7786) (-4.6453, -10.66) knots 0 0 0 0 0.039172 0.079452 0.079452 0.079452 0.079452
  spline S78 degree 3 poles (-4.6453, -10.66) (-4.5588, -10.5479) (-4.3804, -10.3169) (-4.1219, -10.1809) (-3.9887, -10.1108) knots 0 0 0 0 0.041948 0.086488 0.086488 0.086488 0.086488
  spline S79 degree 3 poles (-3.9887, -10.1108) (-3.8388, -10.0537) (-3.5286, -9.9354) (-3.1967, -9.9218) (-3.0252, -9.9147) knots 0 0 0 0 0.047808 0.098905 0.098905 0.098905 0.098905
  spline S80 degree 3 poles (-3.0252, -9.9147) (-2.8153, -9.9201) (-2.4259, -9.9299) (-2.0575, -10.0549) (-1.8878, -10.1126) knots 0 0 0 0 0.062568 0.11604 0.11604 0.11604 0.11604
  spline S81 degree 3 poles (-1.8878, -10.1126) (-1.7437, -10.1859) (-1.4593, -10.3307) (-1.2643, -10.5832) (-1.1681, -10.7077) knots 0 0 0 0 0.047839 0.094429 0.094429 0.094429 0.094429
  spline S82 degree 3 poles (-1.1681, -10.7077) (-1.0914, -10.8456) (-0.9358, -11.1255) (-0.9078, -11.4446) (-0.8936, -11.6064) knots 0 0 0 0 0.046783 0.094914 0.094914 0.094914 0.094914
  circle A0 centre (0, 0) radius 6.2665
  line L77 (3.9578, -56.794) -> (-3.9578, -56.794)
  line L78 (-3.9578, -56.794) -> (-3.9578, -43.206)
  line L79 (-3.9578, -43.206) -> (3.9578, -43.206)
  line L80 (3.9578, -43.206) -> (3.9578, -56.794)
  circle A1 centre (0, 0) radius 61.8943
  line L81 (1.042, -20) -> (1.042, -25)
  line L82 (1.042, -25) -> (0.3632, -25)
  line L83 (0.3632, -25) -> (-2.263, -21.0744)
  line L84 (-2.263, -21.0744) -> (-2.263, -25)
  line L85 (-2.263, -25) -> (-2.8973, -25)
  line L86 (-2.8973, -25) -> (-2.8973, -20)
  line L87 (-2.8973, -20) -> (-2.2186, -20)
  line L88 (-2.2186, -20) -> (0.4076, -23.9291)
  line L89 (0.4076, -23.9291) -> (0.4076, -20)
  line L90 (0.4076, -20) -> (1.042, -20)
  line L91 (18.4908, -21.9611) -> (18.4908, -22.5477)
  line L92 (18.4908, -22.5477) -> (16.3728, -22.5512)
  line L93 (16.3728, -22.5512) -> (16.3728, -20.6958)
  spline S83 degree 3 poles (16.3728, -20.6958) (16.5339, -20.5753) (16.8467, -20.3412) (17.2051, -20.1861) (17.3789, -20.1108) knots 0 0 0 0 0.060121 0.116737 0.116737 0.116737 0.116737
  spline S84 degree 3 poles (17.3789, -20.1108) (17.5525, -20.0536) (17.8983, -19.9397) (18.2619, -19.923) (18.443, -19.9147) knots 0 0 0 0 0.054544 0.108655 0.108655 0.108655 0.108655
  spline S85 degree 3 poles (18.443, -19.9147) (18.6808, -19.9267) (19.1465, -19.9502) (19.573, -20.1382) (19.7817, -20.2302) knots 0 0 0 0 0.070743 0.13857 0.13857 0.13857 0.13857
  spline S86 degree 3 poles (19.7817, -20.2302) (19.9699, -20.3468) (20.345, -20.5791) (20.5757, -20.9552) (20.6907, -21.1426) knots 0 0 0 0 0.065413 0.130387 0.130387 0.130387 0.130387
  spline S87 degree 3 poles (20.6907, -21.1426) (20.7802, -21.3502) (20.9637, -21.7758) (20.9861, -22.2389) (20.9976, -22.4761) knots 0 0 0 0 0.067246 0.137838 0.137838 0.137838 0.137838